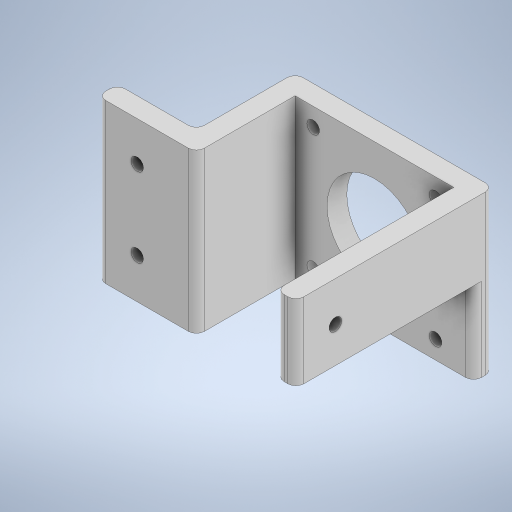
# Autodesk Inventor part: Motor Mount
Saved by Autodesk Inventor 2023.1 (Build 271208000, 208)
## iProperties
Created: 2022-10-30
Part Number: Motor Mount
Material: Generic
Document SubType Name: Modeling
Designer: nicol
Density: 1 g/cm^3
Appearance: Default
Author: nicol
Autodesk Inventor part; units mm, degrees
ref_plane "YZ Plane" through (0, 0, 0) normal (1, 0, 0) x (0, 1, 0)
ref_plane "XZ Plane" through (0, 0, 0) normal (0, 1, 0) x (-1, 0, 0)
ref_plane "XY Plane" through (0, 0, 0) normal (0, 0, 1) x (1, 0, 0)
sketch "Sketch1" plane through (0, 0, 0) normal (0, 0, 1) x (1, 0, 0)
  line L0 (0, 0) -> (40.2, 0)
  line L1 (40.2, 0) -> (40.2, 40.2)
  line L2 (40.2, 40.2) -> (0, 40.2)
  line L3 (0, 40.2) -> (0, 0)
  line L4 (0, 0) -> (5, 0)
  line L5 (40.2, 0) -> (45, 0)
  line L6 (4.6, 35.6) -> (35.6, 35.6) construction
  line L7 (35.6, 35.6) -> (35.6, 4.6) construction
  line L8 (35.6, 4.6) -> (4.6, 4.6) construction
  line L9 (4.6, 4.6) -> (4.6, 35.6) construction
  circle A0 centre (20.1, 20.1) radius 12
  line L10 (0.1, 40.1) -> (40.1, 40.1)
  line L11 (40.1, 40.1) -> (40.1, 0.1)
  line L12 (40.1, 0.1) -> (0.1, 0.1)
  line L13 (0.1, 0.1) -> (0.1, 40.1)
  line L14 (40.2, 40.2) -> (45.2, 40.2)
  line L15 (45.2, 40.2) -> (45.2, 20.1)
  line L16 (45.2, 20.1) -> (40.2, 20.1)
  line L17 (40.2, 20.1) -> (40.2, 40.2)
  line L18 (0, 40.2) -> (-5, 40.2)
  line L19 (-5, 40.2) -> (-5, 0)
  line L20 (-5, 0) -> (0, 0)
  line L21 (0, 0) -> (0, 40.2)
  point P0 (35.6, 20.1)
  point P1 (40.1, 20.1)
  point P2 (20.1, 35.6)
  point P3 (20.1, 40.1)
  point P4 (20.1, 40.2)
  dimension "d0" = 31
  dimension "d1" = 40
  dimension "d5" = 0.1
  dimension "d6" = 0.1
  dimension "d7" = 24
  dimension "d32" = 5
  dimension "d37" = 5
  constraints: 44 end point, 10 parallel, 8 perpendicular, 7 horizontal, 6 midpoint, 4 coincident, 3 vertical alignment, 2 horizontal alignment, 1 centre point, 1 collinear
  measures "d0" distance of L7.end L8.end
  measures "d1" distance of L10.end L11.end
  measures "d5" distance between parallel lines of L0 L12
  measures "d6" distance between parallel lines of L2 L10
  measures "d7" diameter of A0
  measures "d32" distance of L15.end L16.end
  measures "d37" distance of L2.end L18.end
extrude "Extrusion2" add sketch "Sketch1" along normal blind 5 contours L3 L2 L1 L0 | L10 L11 L12 L13
extrude "Extrusion4" add sketch "Sketch1" along normal blind 50 contours L14 L15 L16 L1
extrude "Extrusion5" add sketch "Sketch1" along normal blind 30 contours L20 L19 L18 L3
hole "Hole1" at (4.6, 35.6, 0) at (35.6, 35.6, 0) at (35.6, 4.6, 0) at (4.6, 4.6, 0) direction (0, 0, 1) diameter 3.2 end through all
sketch "Sketch4" plane through (40.2, 40.2, 50) normal (0, 1, 0) x (1, 0, 0)
  line L0 (-45.2, 20) -> (-65.2, 20)
  line L1 (-65.2, 20) -> (-65.2, 25)
  line L2 (-65.2, 25) -> (-45.2, 25)
  line L3 (-45.2, 25) -> (-45.2, 20)
  point P0 (-40.2, 50)
  dimension "d42" = 20
  dimension "d43" = 5
  constraints: 8 end point, 2 parallel, 1 horizontal, 1 perpendicular
  measures "d42" distance of L1.end L2.end
  measures "d43" distance of L0.end L1.end
extrude "Extrusion6" add sketch "Sketch4" against normal up to surface (40.2 mm away)
sketch "Sketch5" plane through (45.2, 20.1, 50) normal (1, 0, 0) x (0, 0, -1)
  line L0 (0, 0) -> (0, 20.1) projected
  line L1 (50, 20.1) -> (0, 20.1) projected
  line L2 (50, 0) -> (0, 0) projected
  point P0 (50, -20.1)
  point P1 (10, 10.05)
  point P2 (49.6, 26)
  point P3 (49.6, 0)
  dimension "d46" = 10
  dimension "d47" = 10.05
  dimension "d48" = 10.05
  constraints: 1 other
  measures "d46" distance from line of L0 point (10, 10.05)
  measures "d48" distance from line of L2 point (10, 10.05)
sketch "Sketch6" plane through (-5, 40.2, 25) normal (0, 0, -1) x (-1, 0, 0)
  line L0 (0, -40.2) -> (20, -40.2) projected
  line L1 (20, 0) -> (20, -40.2) projected
  line L2 (0, 0) -> (20, 0) projected
  line L3 (0, -40.2) -> (0, 0) projected
  point P0 (-5, -40.2)
  point P1 (10, -10)
  point P2 (10, -30)
  point P3 (10, -40.2)
  point P4 (10, 0)
  dimension "d49" = 10
  dimension "d65" = 20
  constraints: 3 vertical alignment, 2 midpoint
  measures "d49" distance from line of L2 point (10, -10)
  measures "d65" distance of point (10, -10) point (10, -30)
hole "Hole3" at (-15, 30.2, 25) at (-15, 10.2, 25) direction (0, 0, 1) diameter 3.2 end through all
hole "Hole4" at (45.2, 30.15, 40) direction (-1, 0, 0) diameter 3.2 end through all
sketch "Sketch7" plane through (40.2, 0, 5) normal (1, 0, 0) x (0, 0, -1)
  line L0 (5, 20.1) -> (0, 20.1) projected
  line L1 (0, 0) -> (0, 20.1) projected
  line L2 (5, 0) -> (0, 0) projected
  line L3 (5, 0) -> (5, 20.1) projected
  point P0 (5, 0)
extrude "Extrusion7" add sketch "Sketch7" along normal blind 5
thicken "Thicken2" operation cut thickness 1 both sides no extend neighbours no toward (0, 1, 0) faces at (41.8667, 20.1, 20)
fillet "Fillet1" radius 2 9 edges at (0, 20.1, 30) (-25, 20.1, 30) (-25, 20.1, 25) (-5, 20.1, 25) (-5, 20.1, 0) (45.2, 20.1, 0) (40.2, 30.65, 50) (45.2, 30.65, 50) (45.2, 10.55, 5)
equation "\"d6\" = d5"
equation "\"d47\" = d48"
body "Solid1"
